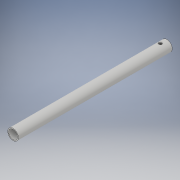
# Autodesk Inventor part: Slanted rod
Saved by Autodesk Inventor 2018 (Build 220112000, 112)
## iProperties
Created: 2018-04-20
Part Number: Slanted rod
Material: Generic
Document SubType Name: Modeling
Designer: 232963
Density: 1 g/cm^3
Appearance: Default
Mass: 32.5516 g
Surface Area: 369.038 cm^2
Volume: 32.5516 cm^3
Author: 232963
Autodesk Inventor part; units mm, degrees
ref_plane "YZ Plane" through (0, 0, 0) normal (1, 0, 0) x (0, 1, 0)
ref_plane "XZ Plane" through (0, 0, 0) normal (0, 1, 0) x (-1, 0, 0)
ref_plane "XY Plane" through (0, 0, 0) normal (0, 0, 1) x (1, 0, 0)
sketch "Sketch2" plane through (0, 0, 0) normal (0, 0, 1) x (1, 0, 0)
  circle A0 centre (0, 0) radius 8.763
  circle A1 centre (0, 0) radius 10.541
  dimension "d4" = 17.526
  dimension "d5" = 1.778
  constraints: 2 centre point, 2 coincident
  measures "d4" diameter of A0
  measures "d5" radial gap between concentric circles of A1 A0
extrude "Extrusion1" add sketch "Sketch2" along normal blind 302.9458
sketch "Sketch3" plane through (0, 0, 0) normal (0, 1, 0) x (-1, 0, 0)
  point P0 (0, 0)
  point P1 (0, 13.2282)
hole "Hole1" at (0, 0, 13.2282) direction (0, -1, 0) diameter 6.35 end through all both
body "Solid1"
